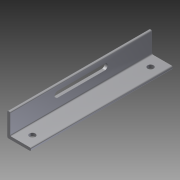
# Autodesk Inventor part: BatteryMountSide
Saved by Autodesk Inventor 2012 (Build 160160000, 160)
## iProperties
Created: 2012-01-09
Part Number: BatteryMountSide
Material: Default
Document SubType Name: Modeling
Designer: William
Density: 1 g/cm^3
Author: William
Autodesk Inventor part; units mm, degrees
ref_plane "YZ Plane" through (0, 0, 0) normal (1, 0, 0) x (0, 1, 0)
ref_plane "XZ Plane" through (0, 0, 0) normal (0, 1, 0) x (-1, 0, 0)
ref_plane "XY Plane" through (0, 0, 0) normal (0, 0, 1) x (1, 0, 0)
sketch "Sketch1" plane through (0, 0, 0) normal (0, 0, 1) x (1, 0, 0)
  line L0 (0, 0) -> (25.4, 0)
  line L1 (25.4, 0) -> (25.4, 3.175)
  line L2 (3.175, 25.4) -> (0, 25.4)
  line L3 (0, 25.4) -> (0, 0)
  line L4 (3.175, 25.4) -> (3.175, 3.175)
  line L5 (3.175, 3.175) -> (25.4, 3.175)
  dimension "d1" = 25.4
  dimension "d2" = 3.175
  dimension "d3" = 3.175
  dimension "d4" = 25.4
  constraints: 12 end point, 2 parallel, 1 horizontal, 1 perpendicular
  measures "d1" distance of L2.end L0.start
  measures "d2" distance between parallel lines of L3 L4
  measures "d3" distance between parallel lines of L0 L5
  measures "d4" distance of L0.start L0.end
extrude "Extrusion1" add sketch "Sketch1" along normal blind 152.4
fillet "Fillet1" radius 1.27 1 edges at (3.175, 25.4, 76.2)
fillet "Fillet2" radius 1.27 5 edges at (0, 25.4, 76.2) (25.4, 3.175, 76.2) (25.4, 0, 76.2) (0, 0, 76.2) (3.175, 3.175, 76.2)
sketch "Sketch2" plane through (4.445, 3.175, 0) normal (0, 1, 0) x (1, 0, 0)
  line L0 (0, -152.4) -> (19.685, -152.4) projected
  line L1 (19.685, 0) -> (0, 0) projected
  circle A0 centre (9.8425, -12.7) radius 3.175
  circle A1 centre (9.8425, -139.7) radius 3.175
  point P0 (-4.445, 0)
  dimension "d9" = 6.35
  dimension "d10" = 6.35
  dimension "d11" = 12.7
  dimension "d12" = 12.7
  constraints: 2 centre point
  measures "d9" diameter of A0
  measures "d10" diameter of A1
  measures "d11" distance from line of L1 A0.centre
  measures "d12" distance from line of A1.centre L0
extrude "Extrusion2" cut sketch "Sketch2" against normal blind 152.4
sketch "Sketch3" plane through (3.175, 24.13, 152.4) normal (1, 0, 0) x (0, 0, -1)
  line L0 (50.8, -4.3683) -> (101.6, -4.3683)
  line L1 (101.6, -10.7183) -> (50.8, -10.7183)
  arc A0 (50.8, -4.3683) -> (50.8, -10.7183) centre (50.8, -7.5433) ccw
  arc A1 (101.6, -10.7183) -> (101.6, -4.3683) centre (101.6, -7.5433) ccw
  point P0 (152.4, -24.13)
  constraints: 4 end point, 4 point on circle, 2 centre point, 1 horizontal, 1 parallel
extrude "Extrusion3" cut sketch "Sketch3" against normal blind 152.4
equation "\"d3\" = d2"
equation "\"d12\" = d11"
body "Solid1"
